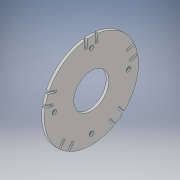
# Autodesk Inventor part: Magnetic Disk
Saved by Autodesk Inventor 2019 (Build 230136000, 136)
## iProperties
Created: 2020-12-02
Part Number: Magnetic Disk
Material: Generic
Document SubType Name: Modeling
Designer: infinity
Density: 1 g/cm^3
Appearance: Default
Author: infinity
Autodesk Inventor part; units mm, degrees
ref_plane "YZ Plane" through (0, 0, 0) normal (1, 0, 0) x (0, 1, 0)
ref_plane "XZ Plane" through (0, 0, 0) normal (0, 1, 0) x (-1, 0, 0)
ref_plane "XY Plane" through (0, 0, 0) normal (0, 0, 1) x (1, 0, 0)
sketch "Sketch1" plane through (0, 0, 0) normal (1, 0, 0) x (0, 1, 0)
  circle A0 centre (0, 0) radius 22.5
  circle A1 centre (0, 0) radius 8.375
  line L0 (8.375, 0) -> (22.5, 0) construction
  line L1 (22.1638, 3.875) -> (7.4246, 3.875) construction
  line L2 (7.4246, -3.875) -> (22.1638, -3.875) construction
  circle A2 centre (17.75, 0) radius 1.0375
  circle A3 centre (0, 17.75) radius 1.0375
  circle A4 centre (-17.75, 0) radius 1.0375
  circle A5 centre (0, -17.75) radius 1.0375
  dimension "d0" = 45
  dimension "d1" = 16.75
  dimension "d2" = 7.75
  dimension "d3" = 3.875
  dimension "d4" = 0
  dimension "d5" = 2.075
  dimension "d6" = 17.75
  dimension "d9" = 360
  constraints: 6 centre point, 6 end point, 6 point on circle, 2 coincident, 2 horizontal, 1 parallel, 1 point on line, 9 other
  measures "d0" diameter of A0
  measures "d1" diameter of A1
  measures "d2" distance between parallel lines of L2 L1
  measures "d3" distance between parallel lines of L0 L1
  measures "d4" distance from line of point (0, 0) L0
  measures "d5" diameter of A2
  measures "d6" distance of point (0, 0) A2.centre
extrude "Extrusion1" add sketch "Sketch1" along normal blind 1
sketch "Sketch2" plane through (0, 0, 0) normal (-1, 0, 0) x (0, 0, 1)
  circle A0 centre (0, 0) radius 8.375 projected
  circle A1 centre (0, 0) radius 22.5 projected
  constraints: 2 centre point
extrude "Extrusion2" add sketch "Sketch2" along normal blind 0.25
sketch "Sketch3" plane through (1, 0, 0) normal (1, 0, 0) x (0, 0, -1)
  line L0 (-3.1, 26.8099) -> (3.1, 26.8099)
  line L1 (3.1, 26.8099) -> (3.1, 18.5)
  line L2 (3.1, 18.5) -> (-3.1, 18.5)
  line L3 (-3.1, 18.5) -> (-3.1, 26.8099)
  circle A0 centre (0, 0) radius 22.5 construction
  line L4 (-2.05, 26.8099) -> (2.05, 26.8099)
  line L5 (2.05, 26.8099) -> (2.05, 18.5)
  line L6 (2.05, 18.5) -> (-2.05, 18.5)
  line L7 (-2.05, 18.5) -> (-2.05, 26.8099)
  line L8 (-26.4557, 5.3365) -> (-24.5398, 11.233)
  line L9 (-24.5398, 11.233) -> (-16.6366, 8.6651)
  line L10 (-16.6366, 8.6651) -> (-18.5525, 2.7685)
  line L11 (-18.5525, 2.7685) -> (-26.4557, 5.3365)
  line L12 (-26.1313, 6.3351) -> (-24.8643, 10.2344)
  line L13 (-24.8643, 10.2344) -> (-16.9611, 7.6665)
  line L14 (-16.9611, 7.6665) -> (-18.228, 3.7671)
  line L15 (-18.228, 3.7671) -> (-26.1313, 6.3351)
  line L16 (-13.2505, -23.5118) -> (-18.2664, -19.8676)
  line L17 (-18.2664, -19.8676) -> (-13.382, -13.1447)
  line L18 (-13.382, -13.1447) -> (-8.3661, -16.7889)
  line L19 (-8.3661, -16.7889) -> (-13.2505, -23.5118)
  line L20 (-14.1, -22.8947) -> (-17.417, -20.4847)
  line L21 (-17.417, -20.4847) -> (-12.5325, -13.7619)
  line L22 (-12.5325, -13.7619) -> (-9.2155, -16.1718)
  line L23 (-9.2155, -16.1718) -> (-14.1, -22.8947)
  line L24 (18.2664, -19.8676) -> (13.2505, -23.5118)
  line L25 (13.2505, -23.5118) -> (8.3661, -16.7889)
  line L26 (8.3661, -16.7889) -> (13.382, -13.1447)
  line L27 (13.382, -13.1447) -> (18.2664, -19.8676)
  line L28 (17.417, -20.4847) -> (14.1, -22.8947)
  line L29 (14.1, -22.8947) -> (9.2155, -16.1718)
  line L30 (9.2155, -16.1718) -> (12.5325, -13.7619)
  line L31 (12.5325, -13.7619) -> (17.417, -20.4847)
  line L32 (24.5398, 11.233) -> (26.4557, 5.3365)
  line L33 (26.4557, 5.3365) -> (18.5525, 2.7685)
  line L34 (18.5525, 2.7685) -> (16.6366, 8.6651)
  line L35 (16.6366, 8.6651) -> (24.5398, 11.233)
  line L36 (24.8643, 10.2344) -> (26.1313, 6.3351)
  line L37 (26.1313, 6.3351) -> (18.228, 3.7671)
  line L38 (18.228, 3.7671) -> (16.9611, 7.6665)
  line L39 (16.9611, 7.6665) -> (24.8643, 10.2344)
  dimension "d15" = 6.2
  dimension "d16" = 3.1
  dimension "d17" = 4
  dimension "d22" = 0
  dimension "d23" = 0
  dimension "d24" = 1.05
  dimension "d25" = 1.05
  dimension "d28" = 360
  constraints: 80 end point, 4 parallel, 2 horizontal, 2 perpendicular, 81 other
  measures "d15" distance of L0.start L0.end
  measures "d16" distance from line of point (0, 0) L3
  measures "d17" distance edge to line of A0 L2
  measures "d22" distance between parallel lines of L0 L4
  measures "d23" distance between parallel lines of L2 L6
  measures "d24" distance between parallel lines of L3 L7
  measures "d25" distance between parallel lines of L1 L5
extrude "Extrusion3" cut sketch "Sketch3" against normal up to surface (1.25 mm away) contours L0 L7 L2 L3 | L0 L1 L2 L5 | L8 L15 L10 L11 | L8 L9 L10 L13 | L16 L23 L18 L19 | L16 L17 L18 L21 | L24 L31 L26 L27 | L24 L25 L26 L29 | L32 L39 L34 L35 | L32 L33 L34 L37
equation "\"d3\" = 0.5 * d2"
equation "\"d16\" = 0.5 * d15"
equation "\"d25\" = d24"
body "Solid1"
